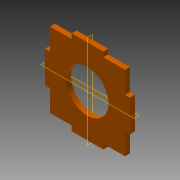
# Autodesk Inventor part: Top
Saved by Autodesk Inventor 2014 SP2 (Build 180246200, 246)
## iProperties
Created: 2014-11-21
Part Number: Top
Material: Generic
Document SubType Name: Modeling
Designer: JLM
Density: 1 g/cm^3
Appearance: Default
Author: JLM
Autodesk Inventor part; units mm, degrees
ref_plane "XY Plane" through (0, 0, 0) normal (0, 0, 1) x (1, 0, 0)
sketch "Sketch1" plane through (0, 0, 0) normal (0, 0, 1) x (1, 0, 0)
  line L0 (-25.5, -25.5) -> (25.5, -25.5)
  line L1 (25.5, -25.5) -> (25.5, 25.5)
  line L2 (25.5, 25.5) -> (-25.5, 25.5)
  line L3 (-25.5, 25.5) -> (-25.5, -25.5)
  line L4 (-25.5, -25.5) -> (25.5, 25.5) construction
  line L5 (25.5, -25.5) -> (-25.5, 25.5) construction
  point P0 (0, 0)
  dimension "d0" = 51
  dimension "d1" = 51
  constraints: 12 end point, 2 midpoint, 2 parallel, 1 horizontal, 1 perpendicular
  measures "d0" distance of L2.end L1.end
  measures "d1" distance of L1.end L0.end
extrude "Extrusion1" add sketch "Sketch1" against normal blind 2.921
sketch "Sketch2" plane through (0, 0, 0) normal (0, 0, 1) x (1, 0, 0)
  line L0 (-25.5, 25.5) -> (-9.5, 25.5)
  line L1 (-9.5, 25.5) -> (-9.5, 22.5)
  line L2 (-9.5, 22.5) -> (-22.5, 22.5)
  line L3 (-25.5, 22.4108) -> (-25.5, 25.5)
  line L4 (-25.5, 25.5) -> (-22.225, 25.5)
  line L5 (-22.5, 22.5) -> (-22.5, 9.5)
  line L6 (-22.5, 9.5) -> (-25.5, 9.5)
  line L7 (-25.5, 9.5) -> (-25.5, 25.5)
  line L8 (25.5, 25.5) -> (-25.5, 25.5) projected
  line L9 (-25.5, 25.5) -> (-25.5, -25.5) projected
  dimension "d59" = 3
  dimension "d62" = 3
  dimension "d67" = 16
  dimension "d73" = 16
  constraints: 16 end point, 4 parallel, 2 collinear, 2 horizontal, 2 perpendicular
  measures "d59" distance of L0.end L1.end
  measures "d62" distance of L5.end L6.end
  measures "d67" distance between parallel lines of L6 L8
  measures "d73" distance from line of L1 L3.start
hole "Hole1" at (-0.1, 0, 0) direction (0, 0, -1) diameter 25.4 end through all
extrude "Extrusion4" cut sketch "Sketch2" against normal up to next
mirror "Mirror1" about plane through (0, 0, 0) normal (1, 0, 0) of "Extrusion4"
mirror "Mirror2" about plane through (0, 0, 0) normal (0, 1, 0) of "Extrusion4", "Mirror1"
equation "\"d1\" = d0"
equation "\"d62\" = d59"
equation "\"d67\" = d73"
equation "\"d53\" = 0.5 * d0"
body "Solid1"
